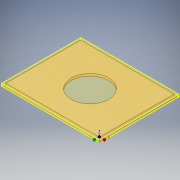
# Autodesk Inventor part: Kettle-Platform
Saved by Autodesk Inventor 2017 (Build 210142000, 142)
## iProperties
Created: 2017-08-30
Part Number: Kettle-Platform
Material: Generic
Document SubType Name: Modeling
Designer: Trent
Density: 1 g/cm^3
Appearance: Yellow Pine - Solid Stained Light Low Gloss
Author: Trent
Autodesk Inventor part; units mm, degrees
ref_plane "YZ Plane" through (0, 0, 0) normal (1, 0, 0) x (0, 1, 0)
ref_plane "XZ Plane" through (0, 0, 0) normal (0, 1, 0) x (-1, 0, 0)
ref_plane "XY Plane" through (0, 0, 0) normal (0, 0, 1) x (1, 0, 0)
sketch "Sketch1" plane through (0, 0, 0) normal (0, 1, 0) x (-1, 0, 0)
  line L0 (-254, 203.2) -> (254, 203.2)
  line L1 (254, 203.2) -> (254, -203.2)
  line L2 (254, -203.2) -> (-254, -203.2)
  line L3 (-254, -203.2) -> (-254, 203.2)
  line L4 (-254, 203.2) -> (254, -203.2) construction
  line L5 (254, 203.2) -> (-254, -203.2) construction
  circle A0 centre (0, 0) radius 101.6
  dimension "d0" = 508
  dimension "d1" = 406.4
  dimension "d2" = 203.2
  constraints: 12 end point, 2 midpoint, 2 parallel, 1 centre point, 1 coincident, 1 horizontal, 1 perpendicular
  measures "d0" distance of L1.end L2.end
  measures "d1" distance of L0.end L1.end
  measures "d2" diameter of A0
extrude "Extrusion1" add sketch "Sketch1" along normal blind 12.7
body "Solid1"
